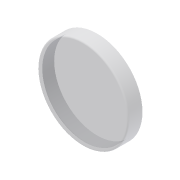
# Autodesk Inventor part: Petri
Saved by Autodesk Inventor 2014 (Build 180170000, 170)
## iProperties
Created: 2015-01-19
Part Number: Petri
Material: Generic
Document SubType Name: Modeling
Designer: Peele
Density: 1 g/cm^3
Appearance: Clear - Light
Author: Peele
Autodesk Inventor part; units mm, degrees
ref_plane "YZ Plane" through (0, 0, 0) normal (1, 0, 0) x (0, 1, 0)
ref_plane "XZ Plane" through (0, 0, 0) normal (0, 1, 0) x (-1, 0, 0)
ref_plane "XY Plane" through (0, 0, 0) normal (0, 0, 1) x (1, 0, 0)
sketch "Sketch1" plane through (0, 0, 0) normal (0, 1, 0) x (-1, 0, 0)
  line L0 (-50, -50) -> (50, -50) construction
  line L1 (50, -50) -> (50, 50) construction
  line L2 (50, 50) -> (-50, 50) construction
  line L3 (-50, 50) -> (-50, -50) construction
  line L4 (-50, -50) -> (50, 50) construction
  line L5 (50, -50) -> (-50, 50) construction
  circle A0 centre (0, 0) radius 60
  dimension "d0" = 100
  dimension "d8" = 120
  constraints: 12 end point, 2 midpoint, 2 parallel, 2 perpendicular, 1 centre point, 1 coincident, 1 horizontal
  measures "d0" distance of L2.end L0.start
  measures "d8" diameter of A0
extrude "Extrusion1" add sketch "Sketch1" along normal blind 2
sketch "Sketch2" plane through (0, 2, 0) normal (0, 1, 0) x (1, 0, 0)
  circle A0 centre (0, 0) radius 60 projected
  circle A1 centre (0, 0) radius 57
  dimension "d9" = 3
  constraints: 1 centre point, 1 coincident
  measures "d9" radial gap between concentric circles of A0 A1
extrude "Extrusion2" add sketch "Sketch2" along normal blind 17
fillet "Fillet1" radius 2 2 edges at (-57, 2, 0) (60, 0, 0)
body "Solid1"
